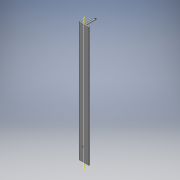
# Autodesk Inventor part: Base_015
Saved by Autodesk Inventor 2016 (Build 200138000, 138)
## iProperties
Created: 2016-11-04
Part Number: Base_015
Material: Generic
Document SubType Name: Modeling
Designer: mattc
Density: 1 g/cm^3
Appearance: Default
Author: mattc
Autodesk Inventor part; units mm, degrees
ref_plane "YZ Plane" through (0, 0, 0) normal (1, 0, 0) x (0, 1, 0)
ref_plane "XZ Plane" through (0, 0, 0) normal (0, 1, 0) x (-1, 0, 0)
ref_plane "XY Plane" through (0, 0, 0) normal (0, 0, 1) x (1, 0, 0)
sketch "Sketch1" plane through (0, 0, 0) normal (0, 1, 0) x (-1, 0, 0)
  line L0 (0, 0) -> (100, 0)
  line L1 (100, 0) -> (100, -1220)
  line L2 (100, -1220) -> (0, -1220)
  line L3 (0, -1220) -> (0, 0)
  dimension "d0" = 100
  dimension "d1" = 1220
  constraints: 8 end point, 2 parallel, 1 horizontal, 1 perpendicular
  measures "d0" distance of L1.end L2.end
  measures "d1" distance of L0.end L1.end
extrude "Extrusion1" add sketch "Sketch1" along normal blind 10
ref_plane "Work Plane1" through (-50, 0, 0) normal (1, 0, 0) x (0, 0, -1)
sketch "Sketch3" plane through (-50, 0, 0) normal (1, 0, 0) x (0, 0, -1)
  line L0 (1220, 0) -> (0, 0) projected
  line L1 (1220, 0) -> (1220, 10) projected
  line L2 (0, 10) -> (1220, 10) projected
  line L3 (0, 0) -> (0, 10) projected
  line L4 (1220, 10) -> (0, 10) projected
  line L5 (0, 10) -> (11.15, 10)
  circle A0 centre (11.15, 120) radius 2.5
  arc A1 (15.15, 120) -> (7.15, 120) centre (11.15, 120) ccw
  line L6 (15.15, 120) -> (15.15, 10)
  line L7 (15.15, 10) -> (7.15, 10)
  line L8 (7.15, 10) -> (7.15, 120)
  dimension "d18" = 11.15
  dimension "d21" = 5
  dimension "d22" = 8
  dimension "d24" = 8
  dimension "d31" = 110
  constraints: 8 end point, 2 centre point, 2 point on circle, 2 point on line, 1 coincident, 1 parallel
  measures "d18" distance of L2.start L5.end
  measures "d21" diameter of A0
  measures "d22" diameter of A1
  measures "d24" distance between parallel lines of L6 L8
  measures "d31" distance of L6.start L6.end
extrude "Extrusion3" add sketch "Sketch3" along normal mid plane 10 contours L2 L8 A1 L6
sketch "Sketch4" plane through (-50, 0, 0) normal (1, 0, 0) x (0, 0, -1)
  arc A0 (15.15, 120) -> (7.15, 120) centre (11.15, 120) ccw projected
  circle A1 centre (11.15, 120) radius 2.5 projected
  line L0 (7.15, 120) -> (7.15, 10) projected
  line L1 (15.15, 124) -> (7.15, 124)
  line L2 (7.15, 124) -> (7.15, 114)
  line L3 (7.15, 114) -> (15.15, 114)
  line L4 (15.15, 114) -> (15.15, 124)
  point P0 (0, 0)
  dimension "d27" = 10
  dimension "d30" = 4
  constraints: 8 end point, 2 parallel, 1 horizontal, 1 perpendicular, 1 point on line
  measures "d27" distance of L2.end L1.end
  measures "d30" distance from line of A0.centre L1
extrude "Extrusion4" cut sketch "Sketch4" along normal mid plane 5
sketch "Sketch5" plane through (0, 10, 0) normal (0, 1, 0) x (1, 0, 0)
  line L0 (-60, 1073.331) -> (-57, 1073.331)
  line L1 (-57, 1073.331) -> (-57, 1093.331)
  line L2 (-57, 1093.331) -> (-60, 1093.331)
  line L3 (-60, 1093.331) -> (-60, 1073.331)
  line L4 (-100, 1220) -> (-100, 0) projected
  line L5 (0, 1220) -> (-100, 1220) projected
  point P0 (0, 0)
  dimension "d32" = 3
  dimension "d33" = 20
  dimension "d34" = 40
  dimension "d35" = 126.669
  constraints: 8 end point, 2 parallel, 1 horizontal, 1 perpendicular
  measures "d32" distance of L2.end L1.end
  measures "d33" distance of L1.end L0.end
  measures "d34" distance between parallel lines of L4 L3
  measures "d35" distance between parallel lines of L5 L2
extrude "Extrusion5" cut sketch "Sketch5" against normal blind 10
body "Solid1"
